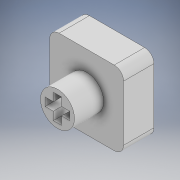
# Autodesk Inventor part: IPC FIX 8
Saved by Autodesk Inventor 2022 (Build 260153000, 153)
## iProperties
Created: 2021-12-31
Part Number: IPC FIX 8
Material: Generic
Document SubType Name: Modeling
Designer: solor
Density: 1 g/cm^3
Appearance: Default
Author: solor
Autodesk Inventor part; units mm, degrees
ref_plane "YZ Plane" through (0, 0, 0) normal (1, 0, 0) x (0, 1, 0)
ref_plane "XZ Plane" through (0, 0, 0) normal (0, 1, 0) x (-1, 0, 0)
sketch "Sketch1" plane through (0, 0, 0) normal (0, 0, 1) x (1, 0, 0)
  line L0 (14.6962, 12.74) -> (14.6962, 0) construction
  line L1 (10.61, 12.2) -> (1.53, 12.2)
  arc A0 (1.53, 12.2) -> (0, 10.67) centre (1.53, 10.67) ccw
  line L2 (0, 10.67) -> (0, 1.53)
  arc A1 (0, 1.53) -> (1.53, 0) centre (1.53, 1.53) ccw
  line L3 (1.53, 0) -> (10.61, 0)
  arc A2 (10.61, 0) -> (12.14, 1.53) centre (10.61, 1.53) ccw
  arc A3 (12.14, 10.67) -> (10.61, 12.2) centre (10.61, 10.67) ccw
  line L4 (12.14, 10.67) -> (12.14, 1.53)
  point P0 (0, 0)
  point P1 (0, 0)
  dimension "d10" = 12.74
  constraints: 10 end point, 8 point on circle, 4 centre point, 2 vertical, 1 point on line
  measures "d10" distance of L0.start L0.end
ref_plane "Work Plane1" through (0, 0, 5) normal (0, 0, 1) x (1, 0, 0)
sketch "Sketch2" plane through (0, 0, 5) normal (0, 0, 1) x (1, 0, 0)
  line L0 (10.88, 12.74) -> (1.8, 12.74) projected
  line L1 (10.88, 12.74) -> (1.8, 12.74) projected
  arc A0 (1.8, 12.74) -> (0, 10.94) centre (1.8, 10.94) ccw projected
  line L2 (0, 10.94) -> (0, 1.8) projected
  arc A1 (0, 1.8) -> (1.8, 0) centre (1.8, 1.8) ccw projected
  line L3 (1.8, 0) -> (10.88, 0) projected
  arc A2 (10.88, 0) -> (12.68, 1.8) centre (10.88, 1.8) ccw projected
  line L4 (12.68, 1.8) -> (12.68, 10.94) projected
  arc A3 (12.68, 10.94) -> (10.88, 12.74) centre (10.88, 10.94) ccw projected
  circle A4 centre (6.34, 6.37) radius 2.8
  line L5 (5.665, 8.395) -> (7.015, 8.395)
  line L6 (7.015, 4.345) -> (5.665, 4.345)
  line L7 (5.665, 4.345) -> (7.015, 8.395) construction
  line L8 (5.665, 8.395) -> (7.015, 4.345) construction
  line L9 (8.365, 5.695) -> (8.365, 7.045)
  line L10 (4.315, 7.045) -> (4.315, 5.695)
  line L11 (4.315, 5.695) -> (8.365, 7.045) construction
  line L12 (8.365, 5.695) -> (4.315, 7.045) construction
  line L13 (4.315, 5.695) -> (5.665, 5.695)
  line L14 (7.015, 5.695) -> (8.365, 5.695)
  line L15 (5.665, 4.345) -> (5.665, 5.695)
  line L16 (5.665, 7.045) -> (5.665, 8.395)
  line L17 (8.365, 7.045) -> (7.015, 7.045)
  line L18 (5.665, 7.045) -> (4.315, 7.045)
  line L19 (7.015, 8.395) -> (7.015, 7.045)
  line L20 (7.015, 5.695) -> (7.015, 4.345)
  point P0 (0, 0)
  dimension "d3" = 5.6
  dimension "d4" = 4.05
  dimension "d5" = 1.35
  dimension "d6" = 4.05
  dimension "d7" = 1.35
  constraints: 32 end point, 10 parallel, 8 perpendicular, 4 midpoint, 2 vertical, 1 centre point
  measures "d3" diameter of A4
  measures "d4" distance of L6.end L5.start
  measures "d5" distance of L5.start L5.end
  measures "d6" distance of L10.end L9.start
  measures "d7" distance of L9.end L9.start
extrude "Extrusion3" add sketch "Sketch1" along normal blind 5
sketch "Sketch3" plane through (0, 0, 5) normal (0, 0, 1) x (1, 0, 0)
  line L0 (10.61, 12.47) -> (1.53, 12.47)
  line L1 (10.61, 12.47) -> (1.53, 12.47)
  arc A0 (1.53, 12.47) -> (-0.27, 10.67) centre (1.53, 10.67) ccw
  line L2 (-0.27, 10.67) -> (-0.27, 1.53)
  arc A1 (-0.27, 1.53) -> (1.53, -0.27) centre (1.53, 1.53) ccw
  line L3 (1.53, -0.27) -> (10.61, -0.27)
  arc A2 (10.61, -0.27) -> (12.41, 1.53) centre (10.61, 1.53) ccw
  line L4 (12.41, 1.53) -> (12.41, 10.67)
  arc A3 (12.41, 10.67) -> (10.61, 12.47) centre (10.61, 10.67) ccw
  circle A4 centre (6.07, 6.1) radius 2.8
  line L5 (5.395, 8.125) -> (6.745, 8.125)
  line L6 (6.745, 4.075) -> (5.395, 4.075)
  line L7 (5.395, 4.075) -> (6.745, 8.125) construction
  line L8 (5.395, 8.125) -> (6.745, 4.075) construction
  line L9 (8.095, 5.425) -> (8.095, 6.775)
  line L10 (4.045, 6.775) -> (4.045, 5.425)
  line L11 (4.045, 5.425) -> (8.095, 6.775) construction
  line L12 (8.095, 5.425) -> (4.045, 6.775) construction
  line L13 (4.045, 5.425) -> (5.395, 5.425)
  line L14 (6.745, 5.425) -> (8.095, 5.425)
  line L15 (5.395, 4.075) -> (5.395, 5.425)
  line L16 (5.395, 6.775) -> (5.395, 8.125)
  line L17 (8.095, 6.775) -> (6.745, 6.775)
  line L18 (5.395, 6.775) -> (4.045, 6.775)
  line L19 (6.745, 8.125) -> (6.745, 6.775)
  line L20 (6.745, 5.425) -> (6.745, 4.075)
  line L21 (10.61, 12.2) -> (1.53, 12.2) projected
  line L22 (0, 10.67) -> (0, 1.53) projected
  point P0 (0, 0)
  point P1 (-0.27, -0.27)
  point P2 (6.07, 12.2)
  point P3 (0, 6.1)
  point P4 (6.07, 6.1)
  dimension "d14" = 5.6
  dimension "d15" = 4.05
  dimension "d16" = 1.35
  dimension "d17" = 4.05
  dimension "d18" = 1.35
  constraints: 42 end point, 10 parallel, 8 perpendicular, 8 point on circle, 6 midpoint, 5 centre point, 2 vertical
  measures "d14" diameter of A4
  measures "d15" distance of L6.end L5.start
  measures "d16" distance of L5.start L5.end
  measures "d17" distance of L10.end L9.start
  measures "d18" distance of L9.end L9.start
extrude "Extrusion4" add sketch "Sketch3" along normal blind 4.8 contours A4
sketch "Sketch4" plane through (0, 0, 0) normal (0, 0, -1) x (-1, 0, 0)
  line L0 (-13.9436, 0) -> (-13.9436, 2.266)
  line L1 (-15.5559, 0) -> (-15.5559, 6.84)
  line L2 (-1.53, 0) -> (-10.61, 0) projected
  line L3 (-9.7626, 9.89) -> (-2.3774, 9.89) construction
  line L4 (-2.3774, 9.89) -> (-2.3774, 6.84) construction
  line L5 (-2.3774, 6.84) -> (-9.7626, 6.84) construction
  line L6 (-9.7626, 6.84) -> (-9.7626, 9.89) construction
  line L7 (-7.4059, 5.4569) -> (-4.7341, 5.4569) construction
  line L8 (-4.7341, 5.4569) -> (-4.7341, 2.266) construction
  line L9 (-4.7341, 2.266) -> (-7.4059, 2.266) construction
  line L10 (-7.4059, 2.266) -> (-7.4059, 5.4569) construction
  line L11 (-7.4047, 9.3092) -> (-8.685, 9.3092)
  line L12 (-8.685, 9.3092) -> (-8.685, 8.7333)
  line L13 (-8.685, 8.7333) -> (-7.506, 8.7333)
  line L14 (-7.506, 8.7333) -> (-7.506, 8.1524)
  line L15 (-7.506, 8.1524) -> (-8.685, 8.1524)
  line L16 (-8.685, 8.1524) -> (-8.685, 6.84)
  line L17 (-8.685, 6.84) -> (-9.4463, 6.84)
  line L18 (-9.4463, 6.84) -> (-9.4463, 9.89)
  line L19 (-9.4463, 9.89) -> (-7.4047, 9.89)
  line L20 (-7.4047, 9.89) -> (-7.4047, 9.3092)
  line L21 (-5.4916, 6.84) -> (-7.1328, 6.84)
  line L22 (-7.1328, 6.84) -> (-7.1328, 7.3714)
  line L23 (-7.1328, 7.3714) -> (-6.6953, 7.3714)
  line L24 (-6.6953, 7.3714) -> (-6.6953, 9.3586)
  line L25 (-6.6953, 9.3586) -> (-7.1328, 9.3586)
  line L26 (-7.1328, 9.3586) -> (-7.1328, 9.89)
  line L27 (-7.1328, 9.89) -> (-5.4916, 9.89)
  line L28 (-5.4916, 9.89) -> (-5.4916, 9.3586)
  line L29 (-5.4916, 9.3586) -> (-5.9291, 9.3586)
  line L30 (-5.9291, 9.3586) -> (-5.9291, 7.3714)
  line L31 (-5.9291, 7.3714) -> (-5.4916, 7.3714)
  line L32 (-5.4916, 7.3714) -> (-5.4916, 6.84)
  line L33 (-2.4021, 6.84) -> (-3.2869, 6.84)
  line L34 (-3.2869, 6.84) -> (-3.8752, 7.8114)
  line L35 (-3.8752, 7.8114) -> (-4.4758, 6.84)
  line L36 (-4.4758, 6.84) -> (-5.3236, 6.84)
  line L37 (-5.3236, 6.84) -> (-4.3324, 8.3749)
  line L38 (-4.3324, 8.3749) -> (-5.284, 9.89)
  line L39 (-5.284, 9.89) -> (-4.3992, 9.89)
  line L40 (-4.3992, 9.89) -> (-3.848, 8.9681)
  line L41 (-3.848, 8.9681) -> (-3.282, 9.89)
  line L42 (-3.282, 9.89) -> (-2.4342, 9.89)
  line L43 (-2.4342, 9.89) -> (-3.3907, 8.407)
  line L44 (-3.3907, 8.407) -> (-2.4021, 6.84)
  spline S0 degree 2 poles (-4.8626, 3.1854) (-4.8626, 2.9902) (-5.0257, 2.6516) (-5.1814, 2.528) knots 0 0 0 1 2 2 2
  spline S1 degree 2 poles (-5.1814, 2.528) (-5.3372, 2.4044) (-5.7845, 2.266) (-6.0737, 2.266) knots 0 0 0 1 2 2 2
  spline S2 degree 2 poles (-6.0737, 2.266) (-6.3827, 2.266) (-6.8449, 2.4069) (-6.9932, 2.528) knots 0 0 0 1 2 2 2
  spline S3 degree 2 poles (-6.9932, 2.528) (-7.139, 2.6491) (-7.2774, 2.9778) (-7.2774, 3.1607) knots 0 0 0 1 2 2 2
  spline S4 degree 2 poles (-7.2774, 3.1607) (-7.2774, 3.4227) (-6.9882, 3.7712) (-6.7139, 3.8874) knots 0 0 0 1 2 2 2
  line L45 (-6.7139, 3.8874) -> (-6.7139, 3.8998)
  spline S5 degree 2 poles (-6.7139, 3.8998) (-6.9833, 4.0307) (-7.1958, 4.404) (-7.1958, 4.6338) knots 0 0 0 1 2 2 2
  spline S6 degree 2 poles (-7.1958, 4.6338) (-7.1958, 4.8019) (-7.0475, 5.096) (-6.9017, 5.2122) knots 0 0 0 1 2 2 2
  spline S7 degree 2 poles (-6.9017, 5.2122) (-6.7608, 5.3234) (-6.3332, 5.4569) (-6.0663, 5.4569) knots 0 0 0 1 2 2 2
  spline S8 degree 2 poles (-6.0663, 5.4569) (-5.7845, 5.4569) (-5.3643, 5.3358) (-5.2284, 5.2369) knots 0 0 0 1 2 2 2
  spline S9 degree 2 poles (-5.2284, 5.2369) (-5.09, 5.138) (-4.9417, 4.8513) (-4.9417, 4.6857) knots 0 0 0 1 2 2 2
  spline S10 degree 2 poles (-4.9417, 4.6857) (-4.9417, 4.4682) (-5.1938, 4.1197) (-5.4533, 3.9986) knots 0 0 0 1 2 2 2
  line L46 (-5.4533, 3.9986) -> (-5.4533, 3.9887)
  spline S11 degree 2 poles (-5.4533, 3.9887) (-5.1493, 3.8651) (-4.8626, 3.4647) (-4.8626, 3.1854) knots 0 0 0 1 2 2 2
  spline S12 degree 2 poles (-5.6189, 3.1533) (-5.6189, 3.3041) (-5.7475, 3.4623) (-5.9551, 3.5636) knots 0 0 0 1 2 2 2
  spline S13 degree 2 poles (-5.9551, 3.5636) (-6.0144, 3.5908) (-6.2393, 3.6773) (-6.3258, 3.7144) knots 0 0 0 1 2 2 2
  spline S14 degree 2 poles (-6.3258, 3.7144) (-6.4049, 3.6353) (-6.531, 3.398) (-6.531, 3.2571) knots 0 0 0 1 2 2 2
  spline S15 degree 2 poles (-6.531, 3.2571) (-6.531, 3.0446) (-6.2591, 2.79) (-6.0391, 2.79) knots 0 0 0 1 2 2 2
  spline S16 degree 2 poles (-6.0391, 2.79) (-5.9773, 2.79) (-5.8241, 2.8295) (-5.7648, 2.8691) knots 0 0 0 1 2 2 2
  spline S17 degree 2 poles (-5.7648, 2.8691) (-5.698, 2.916) (-5.6189, 3.0446) (-5.6189, 3.1533) knots 0 0 0 1 2 2 2
  spline S18 degree 2 poles (-5.6857, 4.5968) (-5.6857, 4.7525) (-5.8908, 4.9378) (-6.0663, 4.9378) knots 0 0 0 1 2 2 2
  spline S19 degree 2 poles (-6.0663, 4.9378) (-6.2344, 4.9378) (-6.4395, 4.7698) (-6.4395, 4.6462) knots 0 0 0 1 2 2 2
  spline S20 degree 2 poles (-6.4395, 4.6462) (-6.4395, 4.5251) (-6.3159, 4.3743) (-6.1849, 4.3125) knots 0 0 0 1 2 2 2
  spline S21 degree 2 poles (-6.1849, 4.3125) (-6.1281, 4.2829) (-5.9699, 4.2211) (-5.8389, 4.1716) knots 0 0 0 1 2 2 2
  spline S22 degree 2 poles (-5.8389, 4.1716) (-5.7598, 4.2754) (-5.6857, 4.4707) (-5.6857, 4.5968) knots 0 0 0 1 2 2 2
  point P0 (0, 0)
  point P1 (-6.07, 0)
  point P2 (-6.07, 2.266)
  point P3 (-6.07, 6.84)
  point P4 (-6.07, 6.84)
  point P5 (-6.07, 2.266)
  dimension "d21" = 2.266
  dimension "d22" = 6.84
  constraints: 4 end point, 3 midpoint, 2 vertical, 4 other
  measures "d21" distance of L0.start L0.end
  measures "d22" distance of L1.start L1.end
extrude "Extrusion5" add sketch "Sketch4" along normal blind 0.9
body "Solid2"
